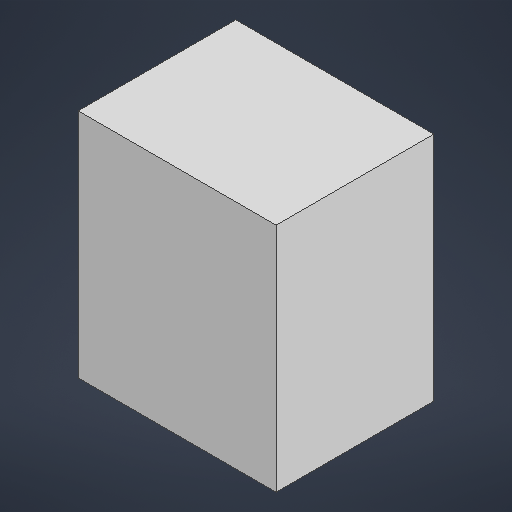
# Autodesk Inventor part: SAFRS-P-0024
Saved by Autodesk Inventor 2026.2 (Build 302298000, 298)
## iProperties
Created: 2025-11-26
Part Number: SAFRS-P-0024
Material: 일반
Document SubType Name: Modeling
Designer: jaewook
Density: 1 g/cm^3
Appearance: 기본값
Author: jaewook
Title: Battery Pack 1
Autodesk Inventor part; units mm, degrees
ref_plane "YZ Plane" through (0, 0, 0) normal (1, 0, 0) x (0, 1, 0)
ref_plane "XZ Plane" through (0, 0, 0) normal (0, 1, 0) x (-1, 0, 0)
ref_plane "XY Plane" through (0, 0, 0) normal (0, 0, 1) x (1, 0, 0)
sketch "스케치1" plane through (0, 0, 0) normal (0, 0, 1) x (1, 0, 0)
  line L0 (28.25, -33) -> (-28.25, -33)
  line L1 (-28.25, -33) -> (-28.25, 33)
  line L2 (-28.25, 33) -> (28.25, 33)
  line L3 (28.25, 33) -> (28.25, -33)
  line L4 (28.25, -33) -> (-28.25, 33) construction
  line L5 (-28.25, -33) -> (28.25, 33) construction
  point P0 (0, 0)
  dimension "d0" = 56.5
  dimension "d1" = 66
  constraints: 12 end point, 2 midpoint, 2 parallel, 1 horizontal, 1 perpendicular
  measures "d0" distance of L1.end L2.end
  measures "d1" distance of L0.end L1.end
extrude "돌출1" add sketch "스케치1" along normal blind 45
